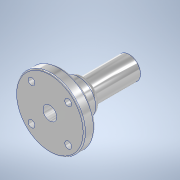
# Autodesk Inventor part: フランジ
Saved by Autodesk Inventor 2020.3 (Build 243373000, 373)
## iProperties
Created: 2020-07-05
Part Number: フランジ
Material: アルミニウム 6061
Document SubType Name: Modeling
Designer: totot
Mass: 14.791 g
Surface Area: 30.442 cm^2
Volume: 5.47815 cm^3
Density: 2.7 g/cm^3
Appearance: アルミニウム - フラット
Author: totot
Autodesk Inventor part; units mm, degrees
ref_plane "YZ Plane" through (0, 0, 0) normal (1, 0, 0) x (0, 1, 0)
ref_plane "XZ Plane" through (0, 0, 0) normal (0, 1, 0) x (-1, 0, 0)
ref_plane "XY Plane" through (0, 0, 0) normal (0, 0, 1) x (1, 0, 0)
sketch "スケッチ1" plane through (0, 0, 0) normal (0, 0, 1) x (1, 0, 0)
  circle A0 centre (0, 0) radius 7.5
  circle A1 centre (0, 0) radius 3
  dimension "d0" = 15
  dimension "d1" = 6
  constraints: 2 centre point, 2 coincident
  measures "d0" diameter of A0
  measures "d1" diameter of A1
extrude "押し出し1" add sketch "スケッチ1" along normal blind 30
sketch "スケッチ2" plane through (0, 0, 30) normal (0, 0, 1) x (1, 0, 0)
  circle A0 centre (0, 0) radius 3
  circle A1 centre (0, 0) radius 15
  dimension "d4" = 6
  dimension "d5" = 30
  constraints: 2 centre point, 2 coincident
  measures "d4" diameter of A0
  measures "d5" diameter of A1
extrude "押し出し2" add sketch "スケッチ2" along normal blind 5
sketch "スケッチ3" plane through (0, 0, 35) normal (0, 0, 1) x (1, 0, 0)
  line L0 (0, 0) -> (8, 0)
  line L1 (8, 0) -> (8, -8)
  line L2 (8, -8) -> (0, -8)
  line L3 (0, -8) -> (0, 0)
  line L4 (8, -8) -> (-8, -8)
  line L5 (-8, -8) -> (-8, 8)
  line L6 (-8, 8) -> (8, 8)
  line L7 (8, 8) -> (8, -8)
  dimension "d8" = 8
  dimension "d9" = 8
  dimension "d10" = 16
  dimension "d11" = 16
  constraints: 16 end point, 4 coincident, 4 parallel, 2 horizontal, 2 perpendicular
  measures "d8" distance of L1.end L2.end
  measures "d9" distance of L0.end L1.end
  measures "d10" distance of L5.end L6.end
  measures "d11" distance of L4.end L5.end
hole "穴1" at (-8, 8, 35) at (8, 8, 35) at (8, -8, 35) at (-8, -8, 35) direction (0, 0, -1) diameter 3 end through all
fillet "フィレット1" radius 2 1 edges at (-7.5, 0, 30)
fillet "フィレット3" radius 1 1 edges at (-15, 0, 30)
sketch "スケッチ4" plane through (0, 0, 0) normal (0, 0, -1) x (-1, 0, 0)
  circle A0 centre (0, 0) radius 3 projected
  circle A1 centre (0, 0) radius 7.5
  circle A2 centre (0, 0) radius 3
  circle A3 centre (0, 0) radius 5
  dimension "d22" = 6
  dimension "d23" = 15
  dimension "d24" = 10
  constraints: 3 centre point, 3 coincident
  measures "d22" diameter of A2
  measures "d23" diameter of A1
  measures "d24" diameter of A3
extrude "押し出し3" cut sketch "スケッチ4" against normal blind 20 contours A1
fillet "フィレット4" radius 2.5 1 edges at (-7.5, 0, 20)
fillet "フィレット5" radius 0.5 2 edges at (5, 0, 0) (-3, 0, 0)
fillet "フィレット6" radius 0.5 1 edges at (-15, 0, 35)
equation "\"d9\" = d8"
equation "\"d10\" = 2 * d9"
equation "\"d11\" = d10"
